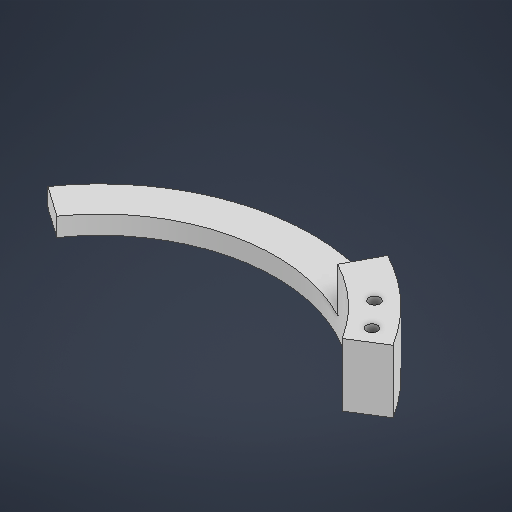
# Autodesk Inventor part: Right_Bottom_Gripper
Saved by Autodesk Inventor 2026.1 (Build 301233020, 233B)
## iProperties
Created: 2025-10-15
Part Number: Right_Bottom_Gripper
Material: Generic
Document SubType Name: Modeling
Designer: Garfieldcmix
Density: 1 g/cm^3
Appearance: Default
Author: Garfieldcmix
Autodesk Inventor part; units mm, degrees
ref_plane "YZ Plane" through (0, 0, 0) normal (1, 0, 0) x (0, 1, 0)
ref_plane "XZ Plane" through (0, 0, 0) normal (0, 1, 0) x (-1, 0, 0)
ref_plane "XY Plane" through (0, 0, 0) normal (0, 0, 1) x (1, 0, 0)
sketch "Sketch1" plane through (0, 0, 0) normal (0, 1, 0) x (-1, 0, 0)
  arc A0 (-40.2823, -25.1712) -> (38.9097, -27.2449) centre (0, 0) ccw
  line L0 (-40.2823, -25.1712) -> (-48.7628, -30.4704)
  line L1 (38.9097, -27.2449) -> (47.1012, -32.9806)
  arc A1 (-48.7628, -30.4704) -> (47.1012, -32.9806) centre (0, 0) ccw
  line L2 (0, -70.4825) -> (0, 11.7471) construction
  dimension "d0" = 47.5
  dimension "d1" = 57.5
  dimension "d2" = 55
  dimension "d3" = 58
  constraints: 4 end point, 4 point on circle, 2 centre point, 2 coincident, 2 line through centre, 1 equal length
  measures "d0" radius of A0
  measures "d1" radius of A1
  measures "d2" angle of L1 L2
  measures "d3" angle of L0 L2
extrude "Extrusion1" add sketch "Sketch1" along normal blind 5
sketch "Sketch2" plane through (0, 5, 0) normal (0, 1, 0) x (1, 0, 0)
  line L0 (40.2823, 25.1712) -> (48.7628, 30.4704) projected
  arc A0 (40.2823, 25.1712) -> (-38.9097, 27.2449) centre (0, 0) ccw projected
  arc A1 (48.7628, 30.4704) -> (-47.1012, 32.9806) centre (0, 0) ccw projected
  line L1 (22.2999, 41.94) -> (26.9946, 50.7695)
  dimension "d6" = 30
  constraints: 2 end point, 2 point on circle, 1 line through centre
  measures "d6" angle of L1 L0
extrude "Extrusion2" add sketch "Sketch2" along normal blind 12
sketch "Sketch3" plane through (0, 17, 0) normal (0, 1, 0) x (1, 0, 0)
  circle A0 centre (41.9284, 31.5953) radius 1.5
  arc A1 (40.2823, 25.1712) -> (22.2999, 41.94) centre (0, 0) ccw construction
  arc A2 (48.7628, 30.4704) -> (26.9946, 50.7695) centre (0, 0) ccw construction
  line L0 (40.2823, 25.1712) -> (48.7628, 30.4704) construction
  line L1 (26.9946, 50.7695) -> (22.2999, 41.94) construction
  line L2 (37.9352, 28.5862) -> (45.9215, 34.6044) construction
  line L3 (32.3949, 34.7393) -> (39.2149, 42.0528) construction
  circle A3 centre (35.8049, 38.3961) radius 1.5
  dimension "d9" = 3
  dimension "d10" = 5
  dimension "d11" = 15
  constraints: 4 end point, 4 point on circle, 2 centre point, 2 line through centre, 2 midpoint, 1 equal radius
  measures "d9" diameter of A0
  measures "d10" angle of L0 L2
  measures "d11" angle of L1 L3
extrude "Extrusion3" cut sketch "Sketch3" against normal up to surface (17 mm away)
body "Solid1"
